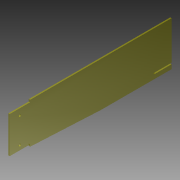
# Autodesk Inventor part: window
Saved by Autodesk Inventor 2014 SP2 (Build 180246200, 246)
## iProperties
Created: 2016-05-05
Part Number: window
Material: Generic
Document SubType Name: Modeling
Designer: cruiser
Density: 1 g/cm^3
Appearance: Clear - Yellow
Author: cruiser
Autodesk Inventor part; units mm, degrees
ref_plane "YZ Plane" through (0, 0, 0) normal (1, 0, 0) x (0, 1, 0)
ref_plane "XZ Plane" through (0, 0, 0) normal (0, 1, 0) x (-1, 0, 0)
ref_plane "XY Plane" through (0, 0, 0) normal (0, 0, 1) x (1, 0, 0)
sketch "Sketch2" plane through (0, 0, 0) normal (1, 0, 0) x (0, 1, 0)
  line L0 (166.1125, -46.875) -> (-166.1125, -46.875)
  line L1 (-166.1125, -46.875) -> (-166.1125, 46.875)
  line L2 (-166.1125, 46.875) -> (166.1125, 46.875)
  line L3 (166.1125, 46.875) -> (166.1125, -46.875)
  line L4 (166.1125, -46.875) -> (-166.1125, 46.875) construction
  line L5 (-166.1125, -46.875) -> (166.1125, 46.875) construction
  line L6 (-166.1125, 41.875) -> (-214.1125, 41.875)
  line L7 (-214.1125, 41.875) -> (-214.1125, -43.7)
  line L8 (-214.1125, -43.7) -> (-166.1125, -43.7)
  line L9 (-166.1125, -43.7) -> (-166.1125, 41.875)
  line L10 (166.1125, -46.875) -> (0, -46.875)
  line L11 (0, -46.875) -> (0, -56.875)
  line L12 (0, -56.875) -> (166.1125, -56.875)
  line L13 (166.1125, -56.875) -> (166.1125, -46.875)
  line L14 (0, 0) -> (0, -46.875)
  line L15 (-166.1125, 46.875) -> (-169.2875, 46.875)
  line L16 (-169.2875, 46.875) -> (-169.2875, 41.875)
  line L17 (-169.2875, 41.875) -> (-166.1125, 41.875)
  line L18 (-166.1125, 41.875) -> (-166.1125, 46.875)
  line L19 (-214.1125, 41.875) -> (-171.6688, 41.875)
  line L20 (-171.6688, 41.875) -> (-171.6688, 46.875)
  line L21 (-171.6688, 46.875) -> (-214.1125, 46.875)
  line L22 (-214.1125, 46.875) -> (-214.1125, 41.875)
  line L23 (-214.1125, 46.875) -> (-173.6687, 46.875)
  line L24 (-173.6687, 46.875) -> (-173.6687, 51.875)
  line L25 (-173.6687, 51.875) -> (-214.1125, 51.875)
  line L26 (-214.1125, 51.875) -> (-214.1125, 46.875)
  line L27 (-171.6688, 46.875) -> (-173.6687, 51.875)
  line L28 (-166.1125, -46.875) -> (0, -46.875)
  line L29 (0, -46.875) -> (0, -48.4625)
  line L30 (0, -48.4625) -> (-166.1125, -48.4625)
  line L31 (-166.1125, -48.4625) -> (-166.1125, -46.875)
  line L32 (0, -56.875) -> (-166.1125, -48.4625)
  dimension "d0" = 332.225
  dimension "d1" = 93.75
  dimension "d6" = 3.175
  dimension "d7" = 5
  dimension "d8" = 48
  dimension "d9" = 10
  dimension "d17" = 0
  dimension "d18" = 3.175
  dimension "d19" = 2.3813
  dimension "d20" = 5
  dimension "d21" = 2
  dimension "d22" = 1.5875
  constraints: 66 end point, 14 parallel, 7 horizontal, 7 perpendicular, 3 midpoint, 2 collinear, 2 point on line
  measures "d0" distance of L1.end L2.end
  measures "d1" distance of L0.end L1.end
  measures "d6" distance between parallel lines of L0 L8
  measures "d7" distance between parallel lines of L2 L6
  measures "d8" distance between parallel lines of L1 L7
  measures "d9" distance between parallel lines of L0 L12
  measures "d17" distance between parallel lines of L14 L11
  measures "d18" distance of L1.end L15.end
  measures "d19" distance between parallel lines of L16 L20
  measures "d20" distance of L25.end L21.end
  measures "d21" distance between parallel lines of L20 L24
  measures "d22" distance between parallel lines of L28 L30
extrude "Extrusion1" add sketch "Sketch2" along normal blind 3.15 contours L13 L12 L11 L0 | L0 L1 L2 L3 | L11 L30 L31 L0 | L11 L32 L30 | L8 L7 L6 L1
sketch "Sketch3" plane through (3.15, 0, 0) normal (1, 0, 0) x (0, 0, -1)
  line L0 (56.875, 0) -> (56.875, 166.1125) projected
  line L1 (56.875, 166.1125) -> (-46.875, 166.1125) projected
  line L2 (43.725, 166.1125) -> (46.875, 166.1125)
  line L3 (46.875, 166.1125) -> (46.875, 126.1125)
  line L4 (46.875, 126.1125) -> (43.725, 126.1125)
  line L5 (43.725, 126.1125) -> (43.725, 166.1125)
  line L6 (-41.875, -166.1125) -> (-41.875, -214.1125) projected
  line L7 (-41.875, -214.1125) -> (43.7, -214.1125) projected
  circle A0 centre (-26.8187, -190.1125) radius 2.5
  line L8 (48.4625, -166.1125) -> (-41.875, -166.1125)
  line L9 (-41.875, -166.1125) -> (-41.875, -214.1125)
  line L10 (-41.875, -214.1125) -> (48.4625, -214.1125)
  line L11 (48.4625, -214.1125) -> (48.4625, -166.1125)
  line L12 (3.2938, -214.1125) -> (3.2938, -166.1125)
  circle A1 centre (33.4063, -190.1125) radius 2.5
  point P0 (0, 0)
  point P1 (-41.875, -169.2875)
  point P2 (-41.875, -171.6688)
  dimension "d11" = 40
  dimension "d12" = 3.15
  dimension "d13" = 10
  dimension "d23" = 5
  dimension "d24" = 24
  dimension "d25" = 30.1125
  constraints: 19 end point, 4 parallel, 2 centre point, 2 horizontal, 2 midpoint, 2 perpendicular, 1 collinear, 1 point on line, 1 symmetric about line, 1 other
  measures "d11" distance of L4.end L2.start
  measures "d12" distance between parallel lines of L3 L5
  measures "d13" distance between parallel lines of L0 L3
  measures "d23" diameter of A0
  measures "d24" distance from line of A0.centre L7
  measures "d25" distance from line of L12 A0.centre
extrude "Extrusion2" cut sketch "Sketch3" against normal blind 10 contours L3 L4 L5 L1 | A0 | A1
equation "\"d0\" = window_z"
equation "\"d1\" = window_y"
equation "\"d6\" = 2 * sm_thickness"
equation "\"d7\" = acrylic_into_frame"
equation "\"d8\" = window_overlap"
equation "\"d9\" = protection_slot_width"
equation "\"d18\" = 2 * sm_thickness"
equation "\"d19\" = 1.5 * sm_thickness"
equation "\"d22\" = sm_thickness"
equation "\"d2\" = clear_acrylic"
equation "\"d11\" = 0.5 * protection_slot_length"
equation "\"d12\" = clear_acrylic"
equation "\"d13\" = protection_slot_width"
equation "\"d23\" = m5_diameter"
equation "\"d24\" = 0.5 * window_overlap"
equation "\"d25\" = 0.333333 * drawer_y"
equation "\"sm_thickness\" = 1.5875"
equation "\"very_thick_acrylic\" = 9.45"
equation "\"thick_acrylic\" = 5.88"
equation "\"thin_acrylic\" = 3.15"
equation "\"clear_acrylic\" = 3.15"
equation "\"wood_thickness\" = 6.72"
equation "\"m3_diameter\" = 3"
equation "\"m4_diameter\" = 4"
equation "\"m5_diameter\" = 5"
equation "\"brass_insert_drill\" = 4"
equation "\"m5_brass_insert_drill\" = 6.7"
equation "\"m3_main_length\" = 14"
equation "\"m3_main_nut_width\" = 5.7"
equation "\"m3_main_nut_thickness\" = 2.5"
equation "\"m3_main_extra\" = 1"
equation "\"stepper_screw_space\" = 35"
equation "\"stepper_shaft_diameter\" = 5"
equation "\"stepper_body_diameter\" = 28"
equation "\"laser_body_diameter\" = 12"
equation "\"carrier_y\" = 251"
equation "\"carrier_z\" = 12"
equation "\"visor_x\" = 253.925"
equation "\"visor_y\" = 85.6"
equation "\"protection_slot\" = 44.2"
equation "\"protection_slot_offset\" = 55.25"
equation "\"window_z\" = 332.225"
equation "\"tray_border\" = 25"
equation "\"bed_z\" = 25"
equation "\"reservoir_x\" = 201"
equation "\"crane_z2\" = 12"
equation "\"tray_y\" = 251"
equation "\"door_sensor\" = 35"
equation "\"linear_bearing_spacing\" = 271"
equation "\"motor_spacing\" = 337"
equation "\"tray_x\" = 251"
equation "\"reservoir_y\" = 201"
equation "\"window_y\" = 93.75"
equation "\"end_stop_spacing\" = 19"
equation "\"window_overlap\" = 48"
equation "\"door_z\" = 332.225"
equation "\"door_x\" = 251"
equation "\"door_overlap\" = 48"
equation "\"acrylic_into_frame\" = 5"
equation "\"protection_slot_width\" = 10"
equation "\"laser_z_offset\" = 55"
equation "\"galvo_frame_x\" = 66"
equation "\"galvo_frame_z\" = 85"
equation "\"laser_y_offset\" = 19.4"
equation "\"thumb_nut_diameter\" = 7"
equation "\"drawer_y\" = 90.3375"
equation "\"frame_total_z\" = 661.5875"
equation "\"printer_z\" = 289"
equation "\"subframe_y_offset\" = 27.5"
equation "\"frame_bottom_z\" = 275"
equation "\"lcd_y\" = 25"
equation "\"drawer_x\" = 257.3"
equation "\"drawer_z\" = 278.175"
equation "\"drawer_z_from_bottom\" = 25"
equation "\"t_galvo_frame\" = 6.72"
equation "\"laser_z\" = 75"
equation "\"nema17_x\" = 43"
equation "\"thumb_nut_offset_y\" = 0"
equation "\"laser_y\" = 15"
equation "\"frame_tilt\" = 1deg"
equation "\"frame_top_z\" = 385"
equation "\"frame_border\" = 48.0375"
equation "\"laser_diameter\" = 12"
equation "\"galvo_frame_y_offset\" = 27.5"
equation "\"lcd_x\" = 72"
equation "\"subframe_x\" = 66"
equation "\"frame_foot_z\" = 12"
equation "\"z_min_from_center\" = 115"
equation "\"m3_press_nut_drill\" = 4.5"
equation "\"m3_head\" = 6"
equation "\"m5_head\" = 10.3"
equation "\"m5_press_nut_drill\" = 6.5"
equation "\"drawer_support_from_top\" = 48"
equation "\"laser_gap\" = 1"
equation "\"frame_screw_from_center\" = 25"
equation "\"drawer_screw_from_center\" = 55"
equation "\"frame_face_y\" = 45"
equation "\"switch_spacing\" = 19"
equation "\"subframe_y\" = 55"
equation "\"al_thickness\" = 1.5875"
equation "\"rivet_diameter\" = 3.3"
equation "\"bend_factor\" = 2.26205"
equation "\"sm_bend\" = 3.591"
equation "\"al_bend\" = 3.591"
equation "\"frame_x\" = 353.375"
equation "\"carrier_z2\" = 25"
equation "\"carrier_y2\" = 76.825"
equation "\"protection_slot_length\" = 80"
body "Solid1"
